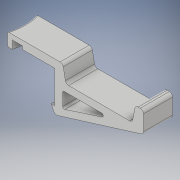
# Autodesk Inventor part: HeadphoneMount
Saved by Autodesk Inventor 2018 (Build 220112000, 112)
## iProperties
Created: 2021-02-09
Part Number: HeadphoneMount
Material: Generic
Document SubType Name: Modeling
Designer: dangl
Density: 1 g/cm^3
Appearance: Default
Author: dangl
Autodesk Inventor part; units mm, degrees
ref_plane "YZ Plane" through (0, 0, 0) normal (1, 0, 0) x (0, 1, 0)
ref_plane "XZ Plane" through (0, 0, 0) normal (0, 1, 0) x (-1, 0, 0)
ref_plane "XY Plane" through (0, 0, 0) normal (0, 0, 1) x (1, 0, 0)
sketch "Sketch1" plane through (0, 0, 0) normal (0, 0, 1) x (1, 0, 0)
  line L0 (0, 7.7456) -> (30, 7.7456)
  line L1 (30, 7.7456) -> (32, -2.2544)
  line L2 (32, -2.2544) -> (73, -2.2544)
  line L3 (73, -2.2544) -> (75, 7.7456)
  line L4 (23, -17.2544) -> (25, -17.2544)
  line L5 (25, -17.2544) -> (25, 2.7456)
  line L6 (25, 2.7456) -> (6, 2.7456)
  line L7 (75, 7.7456) -> (80, 7.7456)
  line L8 (80, 7.7456) -> (80, -5.2544)
  line L9 (80, -5.2544) -> (25, -22.2544)
  line L10 (25, -22.2544) -> (23, -17.2544)
  line L11 (0, 7.7456) -> (0, 2.7456)
  line L12 (0, 2.7456) -> (6, 2.7456)
  point P0 (0, 0)
  dimension "d0" = 20
  dimension "d4" = 5
  dimension "d7" = 2
  dimension "d8" = 10
  dimension "d9" = 45
  dimension "d11" = 41
  dimension "d12" = 2
  dimension "d13" = 5
  dimension "d14" = 13
  dimension "d15" = 5
  dimension "d18" = 0
  dimension "d19" = 6
  dimension "d20" = 30
  dimension "d21" = 25
  dimension "d26" = 2.7456
  dimension "d27" = 2.7456
  constraints: 26 end point, 2 perpendicular, 2 vertical, 1 collinear, 1 horizontal, 1 point on line
  measures "d0" distance of L4.end L5.end
  measures "d4" distance between parallel lines of L0 L6
  measures "d7" distance of L4.start L4.end
  measures "d8" distance between parallel lines of L0 L2
  measures "d9" distance of L3.end L0.end
  measures "d11" distance of L1.end L2.end
  measures "d12" horizontal distance of L1.end L0.end
  measures "d13" distance of L3.end L7.end
  measures "d14" distance of L7.end L8.end
  measures "d15" distance of L4.end L9.end
  measures "d18" distance from line of point (0, 0) L11
  measures "d19" horizontal distance of point (0, 0) L6.end
  measures "d20" horizontal distance of L0.end point (0, 0)
  measures "d21" distance from line of point (0, 0) L5
  measures "d26" distance from line of point (0, 0) L6
  measures "d27" distance of point (0, 0) L11.end
extrude "Extrusion1" add sketch "Sketch1" along normal mid plane 18
sketch "Sketch4" plane through (0, 2.7456, 9) normal (0, -1, 0) x (1, 0, 0)
  arc A0 (-1.1431, -18) -> (-1.1431, 0) centre (-36, -9) ccw
  line L0 (0, 0) -> (0, -18) projected
  arc A1 (5.0244, -18) -> (5.0244, 0) centre (-36, -9) ccw
  arc A2 (-4.251, -18) -> (-4.251, 0) centre (-36, -9) ccw
  line L1 (30, 0) -> (0, 0) projected
  line L2 (5.0244, 0) -> (-4.251, 0)
  line L3 (0, -18) -> (30, -18) projected
  line L4 (5.0244, -18) -> (-4.251, -18)
  point P0 (0, -9)
  dimension "d28" = 72
  dimension "d29" = 36
  dimension "d30" = 84
  dimension "d31" = 66
  constraints: 6 point on circle, 4 end point, 4 point on line, 3 centre point, 2 coincident, 2 collinear
  measures "d28" diameter of A0
  measures "d29" distance from line of L0 A0.centre
  measures "d30" diameter of A1
  measures "d31" diameter of A2
extrude "Extrusion2" add sketch "Sketch4" against normal blind 5
extrude "Extrusion3" add sketch "Sketch4" along normal blind 3 contours L4 A2 L2 A0
extrude "Extrusion4" cut sketch "Sketch4" against normal blind 2 contours A0 L0 L4 | A0 L2 L0 | L0 L1 A1 L3
fillet "Fillet1" radius 2 2 edges at (30, 7.7456, 0) (75, 7.7456, 0)
fillet "Fillet2" radius 2 5 edges at (73, -2.2544, 0) (32, -2.2544, 0) (25, -22.2544, 0) (80, -5.2544, 0) (80, 7.7456, 0)
fillet "Fillet3" radius 1 2 edges at (-3, 7.7456, 0) (-3, -0.2544, 0)
sketch "Sketch5" plane through (0, 0, 9) normal (0, 0, 1) x (1, 0, 0)
  line L0 (30, -6.7544) -> (60.4607, -6.7544)
  line L1 (60.4607, -6.7544) -> (30, -16.6287)
  line L2 (30, -16.6287) -> (30, -6.7544)
  line L3 (71.3604, -2.2544) -> (33.6396, -2.2544) projected
  line L4 (26.7625, -21.7097) -> (78.5906, -5.6901) projected
  line L5 (25, 2.7456) -> (25, -17.2544) projected
  point P0 (0, 0)
  dimension "d41" = 4.5
  dimension "d42" = 0.785
  dimension "d43" = 5
  constraints: 6 end point, 1 horizontal, 1 perpendicular
  measures "d41" distance between parallel lines of L3 L0
  measures "d42" angle of L4 L1
  measures "d43" distance between parallel lines of L5 L2
extrude "Extrusion5" cut sketch "Sketch5" against normal through all
fillet "Fillet4" radius 1 3 edges at (60.4607, -6.7544, 0) (30, -6.7544, 0) (30, -16.6287, 0)
equation "\"d29\" = 0.5 * d28"
body "Solid1"
